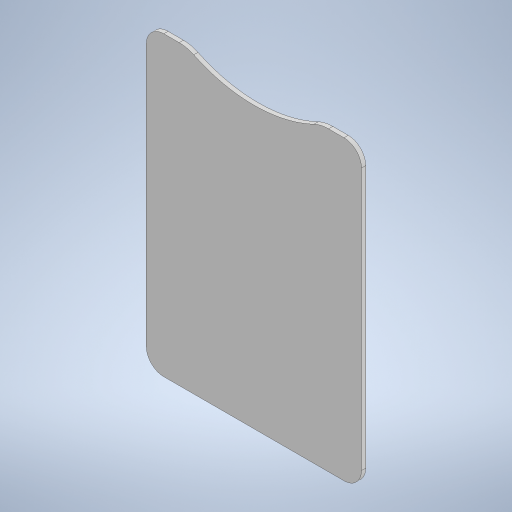
# Autodesk Inventor part: cover
Saved by Autodesk Inventor 2023.2 (Build 272271000, 271)
## iProperties
Created: 2022-12-26
Part Number: cover
Material: Generic
Document SubType Name: Modeling
Designer: omrfrkmll
Density: 1 g/cm^3
Appearance: Default
Author: omrfrkmll
Autodesk Inventor part; units mm, degrees
ref_plane "YZ Plane" through (0, 0, 0) normal (1, 0, 0) x (0, 1, 0)
ref_plane "XZ Plane" through (0, 0, 0) normal (0, 1, 0) x (-1, 0, 0)
ref_plane "XY Plane" through (0, 0, 0) normal (0, 0, 1) x (1, 0, 0)
sketch "Sketch1" plane through (0, 0, 0) normal (0, 0, 1) x (1, 0, 0)
  line L0 (-63.6219, 46.5321) -> (-63.6219, -113.4679)
  line L1 (-63.6219, -113.4679) -> (-63.6219, 46.5321)
  arc A0 (-53.6219, 56.5321) -> (-63.6219, 46.5321) centre (-53.6219, 46.5321) ccw
  arc A1 (-35.6399, 54.6078) -> (-44.1996, 56.5321) centre (-44.1996, 36.5321) ccw
  line L2 (-53.6219, 56.5321) -> (-44.1996, 56.5321)
  arc A2 (46.9558, 56.5321) -> (38.396, 54.6078) centre (46.9558, 36.5321) ccw
  line L3 (56.3781, 56.5321) -> (46.9558, 56.5321)
  line L4 (46.9558, 56.5321) -> (56.3781, 56.5321)
  line L5 (66.3781, -113.4679) -> (66.3781, 46.5321)
  line L6 (66.3781, 46.5321) -> (66.3781, -113.4679)
  arc A3 (56.3781, -123.4679) -> (66.3781, -113.4679) centre (56.3781, -113.4679) ccw
  line L7 (56.3781, -123.4679) -> (-53.6219, -123.4679)
  arc A4 (-63.6219, -113.4679) -> (-53.6219, -123.4679) centre (-53.6219, -113.4679) ccw
  arc A5 (-63.6219, -113.4679) -> (-53.6219, -123.4679) centre (-53.6219, -113.4679) ccw
  arc A6 (-53.6219, 56.5321) -> (-63.6219, 46.5321) centre (-53.6219, 46.5321) ccw
  arc A7 (-35.6399, 54.6078) -> (38.396, 54.6078) centre (1.3781, 132.779) ccw
  arc A8 (-35.6399, 54.6078) -> (38.396, 54.6078) centre (1.3781, 132.779) ccw
  arc A9 (66.3781, 46.5321) -> (56.3781, 56.5321) centre (56.3781, 46.5321) ccw
  arc A10 (56.3781, -123.4679) -> (66.3781, -113.4679) centre (56.3781, -113.4679) ccw
  arc A11 (66.3781, 46.5321) -> (56.3781, 56.5321) centre (56.3781, 46.5321) ccw
  arc A12 (-35.6399, 54.6078) -> (-44.1996, 56.5321) centre (-44.1996, 36.5321) ccw
  arc A13 (46.9558, 56.5321) -> (38.396, 54.6078) centre (46.9558, 36.5321) ccw
  line L8 (-53.6219, -123.4679) -> (56.3781, -123.4679)
  line L9 (-53.6219, -123.4679) -> (56.3781, -123.4679)
  line L10 (-61.6219, -113.4679) -> (-61.6219, 46.5321)
  arc A14 (-53.6219, 54.5321) -> (-61.6219, 46.5321) centre (-53.6219, 46.5321) ccw
  line L11 (-53.6219, 54.5321) -> (-44.1996, 54.5321)
  arc A15 (-36.4958, 52.8002) -> (-44.1996, 54.5321) centre (-44.1996, 36.5321) ccw
  arc A16 (-36.4958, 52.8002) -> (39.252, 52.8002) centre (1.3781, 132.779) ccw
  arc A17 (46.9558, 54.5321) -> (39.252, 52.8002) centre (46.9558, 36.5321) ccw
  line L12 (46.9558, 54.5321) -> (56.3781, 54.5321)
  arc A18 (64.3781, 46.5321) -> (56.3781, 54.5321) centre (56.3781, 46.5321) ccw
  line L13 (64.3781, 46.5321) -> (64.3781, -113.4679)
  arc A19 (56.3781, -121.4679) -> (64.3781, -113.4679) centre (56.3781, -113.4679) ccw
  line L14 (56.3781, -121.4679) -> (-53.6219, -121.4679)
  arc A20 (-61.6219, -113.4679) -> (-53.6219, -121.4679) centre (-53.6219, -113.4679) ccw
  arc A21 (-53.6219, 57.2321) -> (-64.3219, 46.5321) centre (-53.6219, 46.5321) ccw
  line L15 (-53.6219, 57.2321) -> (-44.1996, 57.2321)
  arc A22 (-35.3403, 55.2404) -> (-44.1996, 57.2321) centre (-44.1996, 36.5321) ccw
  arc A23 (-35.3403, 55.2404) -> (38.0964, 55.2404) centre (1.3781, 132.779) ccw
  arc A24 (46.9558, 57.2321) -> (38.0964, 55.2404) centre (46.9558, 36.5321) ccw
  line L16 (-64.3219, 46.5321) -> (-64.3219, -113.4679)
  line L17 (56.3781, 57.2321) -> (46.9558, 57.2321)
  arc A25 (67.0781, 46.5321) -> (56.3781, 57.2321) centre (56.3781, 46.5321) ccw
  line L18 (67.0781, -113.4679) -> (67.0781, 46.5321)
  arc A26 (56.3781, -124.1679) -> (67.0781, -113.4679) centre (56.3781, -113.4679) ccw
  line L19 (56.3781, -124.1679) -> (-53.6219, -124.1679)
  arc A27 (-64.3219, -113.4679) -> (-53.6219, -124.1679) centre (-53.6219, -113.4679) ccw
  line L20 (-60.9219, 46.5321) -> (-60.9219, -113.4679)
  arc A28 (-60.9219, -113.4679) -> (-53.6219, -120.7679) centre (-53.6219, -113.4679) ccw
  line L21 (-53.6219, -120.7679) -> (56.3781, -120.7679)
  arc A29 (56.3781, -120.7679) -> (63.6781, -113.4679) centre (56.3781, -113.4679) ccw
  line L22 (63.6781, -113.4679) -> (63.6781, 46.5321)
  arc A30 (63.6781, 46.5321) -> (56.3781, 53.8321) centre (56.3781, 46.5321) ccw
  line L23 (56.3781, 53.8321) -> (46.9558, 53.8321)
  arc A31 (46.9558, 53.8321) -> (39.5516, 52.1675) centre (46.9558, 36.5321) ccw
  arc A32 (-36.7954, 52.1675) -> (39.5516, 52.1675) centre (1.3781, 132.779) ccw
  arc A33 (-36.7954, 52.1675) -> (-44.1996, 53.8321) centre (-44.1996, 36.5321) ccw
  line L24 (-44.1996, 53.8321) -> (-53.6219, 53.8321)
  arc A34 (-53.6219, 53.8321) -> (-60.9219, 46.5321) centre (-53.6219, 46.5321) ccw
  point P0 (0, 0)
  point P1 (1.3781, -33.4679)
  dimension "d0" = 2
  dimension "d1" = 0.7
  dimension "d2" = 0.7
  dimension "d3" = 0.7
  dimension "d4" = 0.7
  dimension "d5" = 0.7
  dimension "d6" = 0.7
  dimension "d7" = 0.7
  dimension "d8" = 0.7
  dimension "d11" = 0.7
  constraints: 70 point on circle, 50 end point, 35 centre point, 7 equal length, 5 coincident, 4 tangent, 3 point on line, 2 horizontal, 1 concentric, 1 vertical, 26 other
  measures "d0" distance between parallel lines of L0 L10
  measures "d1" radial gap between concentric circles of A0 A21
  measures "d2" distance between parallel lines of L0 L16
  measures "d3" distance between parallel lines of L3 L17
  measures "d4" radial gap between concentric circles of A9 A25
  measures "d5" distance between parallel lines of L5 L18
  measures "d6" radial gap between concentric circles of A3 A26
  measures "d7" distance between parallel lines of L7 L19
  measures "d8" radial gap between concentric circles of A4 A27
  measures "d11" radial gap between concentric circles of A14 A34
extrude "Extrusion1" add sketch "Sketch1" along normal blind 0.6 contours A0 L2 A1 A7 A2 L3 A9 L5 A3 L7 A4 L0 | L10 A14 L11 A15 A16 A17 L12 A18 L13 A19 L14 A20 | L15 A22 A23 A24 L17 A25 L18 A26 L19 A27 L16 A21 | A34 L24 A33 A32 A31 L23 A30 L22 A29 L21 A28 L20
extrude "Extrusion2" add sketch "Sketch1" against normal blind 2
body "Solid1"
